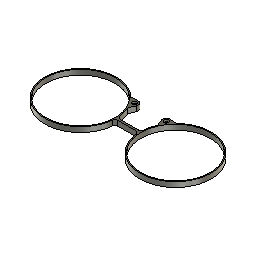
Prop Guard Back v17 (Autodesk Fusion 360 design; units mm, degrees)
Autodesk Fusion 360 part; units mm, degrees
sketch "Sketch1" plane through (0, 0, 0) normal (0, 0, 1) x (1, 0, 0)
  line L0 (25, 40) -> (-25, 40)
  line L1 (-25, 40) -> (-25, -40)
  line L2 (-25, -40) -> (25, -40)
  line L3 (25, -40) -> (25, 40)
  line L4 (25, 40) -> (-25, -40) construction
  line L5 (-25, 40) -> (25, -40) construction
  line L6 (25, 40) -> (46.6506, 52.5)
  line L7 (25, 40) -> (55, 40) construction
  line L8 (0, 40) -> (0, -40)
  line L9 (-25, 0) -> (25, 0)
  line L10 (25, 40) -> (23.5, 42.5981)
  line L11 (23.5, 42.5981) -> (45.1506, 55.0981)
  line L12 (45.1506, 55.0981) -> (46.6506, 52.5)
  line L13 (25, 40) -> (26.5, 37.4019)
  line L14 (26.5, 37.4019) -> (48.1506, 49.9019)
  line L15 (23.5, 42.5981) -> (19, 40)
  line L16 (26.5, 37.4019) -> (25, 36.5359)
  line L17 (48.1506, 49.9019) -> (46.6506, 52.5)
  circle A0 centre (46.6506, 52.5) radius 12
  circle A1 centre (46.6506, 52.5) radius 10
  line L18 (46.6506, 52.5) -> (41.6506, 61.1603)
  line L19 (46.6506, 52.5) -> (55.3109, 57.5)
  line L20 (46.6506, 52.5) -> (51.6506, 43.8397)
  circle A2 centre (46.6506, 52.5) radius 1.5
  line L21 (46.6506, 52.5) -> (51.8468, 55.5)
  line L22 (46.6506, 52.5) -> (43.6506, 57.6962)
  circle A3 centre (-46.6506, 52.5) radius 1.5
  line L23 (-23.5, 42.5981) -> (-45.1506, 55.0981)
  line L24 (-26.5, 37.4019) -> (-48.1506, 49.9019)
  circle A4 centre (-46.6506, 52.5) radius 12
  circle A5 centre (-46.6506, 52.5) radius 10
  line L25 (-26.5, 37.4019) -> (-25, 36.5359)
  line L26 (-23.5, 42.5981) -> (-19, 40)
  circle A6 centre (-46.6506, -52.5) radius 10
  line L27 (-26.5, -37.4019) -> (-48.1506, -49.9019)
  line L28 (-23.5, -42.5981) -> (-45.1506, -55.0981)
  line L29 (-23.5, -42.5981) -> (-19, -40)
  line L30 (-26.5, -37.4019) -> (-25, -36.5359)
  line L31 (23.5, -42.5981) -> (19, -40)
  line L32 (26.5, -37.4019) -> (25, -36.5359)
  line L33 (26.5, -37.4019) -> (48.1506, -49.9019)
  line L34 (23.5, -42.5981) -> (45.1506, -55.0981)
  circle A7 centre (46.6506, -52.5) radius 12
  circle A8 centre (46.6506, -52.5) radius 10
  circle A9 centre (46.6506, -52.5) radius 1.5
  circle A10 centre (-46.6506, -52.5) radius 10
  circle A11 centre (-46.6506, -52.5) radius 12
  line L35 (25, 0) -> (25, -40)
  line L36 (0, 0) -> (0, -9)
  line L37 (0, -9) -> (0, -10.6)
  line L38 (0, -9) -> (0, -7.4)
  line L39 (0, -10.6) -> (14, -10.6)
  line L40 (0, -9) -> (1, -9)
  line L41 (0, -7.4) -> (14, -7.4)
  line L42 (14, -10.6) -> (14, -7.4)
  line L43 (-14, -10.6) -> (-14, -7.4)
  line L44 (0, -7.4) -> (-14, -7.4)
  line L45 (0, -10.6) -> (-14, -10.6)
  line L46 (0, 7.4) -> (-14, 7.4)
  line L47 (-14, 10.6) -> (-14, 7.4)
  line L48 (0, 10.6) -> (-14, 10.6)
  line L49 (0, 10.6) -> (14, 10.6)
  line L50 (0, 7.4) -> (14, 7.4)
  line L51 (14, 10.6) -> (14, 7.4)
  line L52 (19, -40) -> (25.9282, -44)
  line L53 (25, -36.5359) -> (25, -31.5359)
  line L54 (19, -40) -> (16, -40)
  line L55 (14.6699, -37.5) -> (34.8771, -37.5) construction
  circle A12 centre (46.6506, -52.5) radius 35
  circle A13 centre (46.6506, -52.5) radius 34
  circle A14 centre (-46.6506, -52.5) radius 35
  circle A15 centre (-46.6506, -52.5) radius 34
  circle A16 centre (-46.6506, 52.5) radius 35
  circle A17 centre (-46.6506, 52.5) radius 34
  circle A18 centre (46.6506, 52.5) radius 35
  circle A19 centre (46.6506, 52.5) radius 34
  line L56 (46.6506, -52.5) -> (46.6506, 52.5)
  line L57 (46.6506, -52.5) -> (-46.6506, -52.5)
  line L58 (46.6506, -52.5) -> (46.6506, -53.5)
  line L59 (-46.6506, -52.5) -> (-46.6506, -53.5)
  line L60 (-46.6506, -53.5) -> (46.6506, -53.5)
  line L61 (46.6506, -52.5) -> (46.6506, -51.5)
  line L62 (-46.6506, -51.5) -> (46.6506, -51.5)
  line L63 (-46.6506, -52.5) -> (-46.6506, -51.5)
  line L64 (-46.6506, 53.5) -> (46.6506, 53.5)
  line L65 (-46.6506, 51.5) -> (46.6506, 51.5)
  line L66 (46.6506, 0) -> (47.1506, 0)
  line L67 (47.1506, 0) -> (47.1506, -17.5036)
  line L68 (47.1506, 0) -> (47.1506, 17.5036)
  line L69 (46.1506, 0) -> (46.1506, 17.5036)
  line L70 (46.1506, 0) -> (46.1506, -17.5036)
  line L71 (-46.1506, 0) -> (-46.1506, 17.5036)
  line L72 (-47.1506, 0) -> (-47.1506, 17.5036)
  line L73 (-47.1506, 0) -> (-47.1506, -17.5036)
  line L74 (-46.1506, 0) -> (-46.1506, -17.5036)
  line L75 (-47.1506, 0) -> (60, 0)
  line L76 (25, -40) -> (25, -30.5)
  line L77 (25, -30.5) -> (15.5, -30.5)
  circle A20 centre (15.5, -30.5) radius 1.2
  circle A21 centre (15.5, -30.5) radius 3.6
  circle A22 centre (-15.5, -30.5) radius 3.6
  circle A23 centre (-15.5, -30.5) radius 1.2
  line L78 (15.5, -30.5) -> (15.5, -29.3)
  circle A24 centre (15.5, -30.5) radius 2.2
  circle A25 centre (-15.5, -30.5) radius 2.2
  point P0 (-46.6506, -52.5)
  dimension "d1" = 50
  dimension "d2" = 80
  dimension "d4" = 25
  dimension "d5" = 30
  dimension "d6" = 3
  dimension "d7" = 25
  dimension "d8" = 24
  dimension "d9" = 20
  dimension "d10" = 3
  dimension "d11" = 6
  dimension "d13" = 6
  dimension "d23" = 9
  dimension "d24" = 1.6
  dimension "d25" = 1.6
  dimension "d26" = 14
  dimension "d51" = 8
  dimension "d76" = 5
  dimension "d77" = 3
  dimension "d88" = 5
  dimension "d130" = 70
  dimension "d131" = 68
  dimension "d132" = 1
  dimension "d133" = 0.5
  dimension "d140" = 9.5
  dimension "d141" = 9.5
  dimension "d142" = 2.4
  dimension "d143" = 7.2
  dimension "d147" = 4.4
  constraint horizontal L0
  constraint perpendicular L0 L1
  constraint parallel L0 L2
  constraint parallel L1 L3
  constraint coincident L4 L36.start
  constraint coincident L5 L36.start
  constraint coincident L36.start origin
  constraint horizontal L7
  constraint midpoint L0 L8.start
  constraint midpoint L2 L8.end
  constraint midpoint L1 L9.start
  constraint midpoint L3 L9.end
  constraint perpendicular L6 L10
  constraint perpendicular L10 L11
  constraint symmetric L0.start L6 L3.end
  constraint symmetric L6 L10.end L13.end
  constraint symmetric L6 L11.end L14.end
  constraint coincident L0 L15.end
  constraint perpendicular L10 L15
  constraint coincident L3 L16.end
  constraint perpendicular L13 L16
  constraint symmetric L12.end L6 L17.end
  constraint coincident L6.end L12.end
  constraint concentric A0 A1
  constraint coincident A1 L18.end
  constraint parallel L12 L18
  constraint coincident A1 L19.end
  constraint perpendicular L12 L19
  constraint coincident A1 L20.end
  constraint perpendicular L19 L20
  constraint perpendicular L20 L21
  constraint parallel L18 L22
  constraint symmetric L8 L10.end L23.start
  constraint symmetric L8 L11.end L23.end
  constraint symmetric L8 L13.end L24.start
  constraint symmetric L8 L14.end L24.end
  constraint symmetric L8 L15.end L26.end
  constraint symmetric L8 L16.end L25.end
  constraint symmetric L8 A0 A4
  constraint symmetric L8 A1 A5
  constraint symmetric L8 A2 A3
  constraint symmetric L9 L10.end L31.start
  constraint symmetric L9 L11.end L34.end
  constraint symmetric L9 L13.end L32.start
  constraint symmetric L9 L14.end L33.end
  constraint symmetric L9 L15.end L31.end
  constraint symmetric L9 L16.end L32.end
  constraint symmetric L9 A0 A7
  constraint symmetric L9 A1 A8
  constraint symmetric L9 A2 A9
  constraint symmetric L9 L23.start L28.start
  constraint symmetric L9 L23.end L28.end
  constraint symmetric L9 L24.start L27.start
  constraint symmetric L9 L24.end L27.end
  constraint symmetric L9 A3.centre P0
  constraint symmetric L9 A5 A6
  constraint symmetric L9 L25.end L30.end
  constraint symmetric L9 L26.end L29.end
  constraint symmetric L9 A5 A10
  constraint symmetric L9 A4 A11
  constraint perpendicular L9 L36
  constraint parallel L8 L37
  constraint parallel L36 L38
  constraint perpendicular L37 L39
  constraint perpendicular L38 L40
  constraint symmetric L37.end L40 L38.end
  constraint symmetric L39.end L40 L41.end
  constraint symmetric L8 L37.end L39.start
  constraint symmetric L8 L39.end L43.start
  constraint symmetric L8 L38.end L41.start
  constraint symmetric L8 L41.end L43.end
  constraint symmetric L9 L37.end L48.start
  constraint symmetric L9 L39.end L49.end
  constraint symmetric L9 L38.end L46.start
  constraint symmetric L9 L41.end L50.end
  constraint symmetric L9 L43.start L47.start
  constraint symmetric L9 L43.end L46.end
  constraint parallel L34 L52
  constraint parallel L2 L54
  constraint horizontal L55
  constraint concentric A8 A12
  constraint concentric A9 A13
  constraint symmetric L8 A12 A14
  constraint symmetric L8 A13 A15
  constraint symmetric L9 A12 A18
  constraint symmetric L9 A13 A19
  constraint symmetric L9 A14 A16
  constraint symmetric L9 A15 A17
  constraint coincident A7.centre A8.centre
  constraint coincident P0 A6.centre
  constraint perpendicular L57 L58
  constraint symmetric L8 A7.centre P0
  constraint symmetric L8 L58.end L59.end
  constraint symmetric L57 A7.centre A8.centre
  constraint symmetric L57 L58.end L61.end
  constraint symmetric L57 P0 A6.centre
  constraint symmetric L57 L59.end L62.start
  constraint symmetric L9 L58.end L64.end
  constraint symmetric L9 L59.end L64.start
  constraint symmetric L9 L61.end L65.end
  constraint symmetric L9 L62.start L65.start
  constraint midpoint L56 L66.start
  constraint perpendicular L56 L66
  constraint coincident A12 L67.end
  constraint perpendicular L66 L67
  constraint coincident A18 L68.end
  constraint perpendicular L66 L68
  constraint symmetric L56 L66.end L69.start
  constraint symmetric L56 L67.end L70.end
  constraint symmetric L56 L68.end L69.end
  constraint symmetric L8 L66.end L72.start
  constraint symmetric L8 L67.end L73.end
  constraint symmetric L8 L68.end L72.end
  constraint symmetric L8 L69.start L71.start
  constraint symmetric L8 L69.end L71.end
  constraint symmetric L8 L70.end L74.end
  constraint perpendicular L71 L75
  constraint perpendicular L2 L76
  constraint perpendicular L35 L77
  constraint coincident L77.end A20.centre
  constraint concentric A20 A21
  constraint symmetric L8 A20 A23
  constraint symmetric L8 A21 A22
  constraint coincident A20 L78.end
  constraint perpendicular L77 L78
  constraint concentric A20 A24
  constraint symmetric L8 A24 A25
  measures "d1" distance of L1.end L2.end
  measures "d2" distance of L0.end L1.end
  measures "d4" distance of L0.start L6.end
  measures "d5" angle of L6 L7
  measures "d6" distance of L0.start L10.end
  measures "d7" distance of L10.end L11.end
  measures "d8" diameter of A0
  measures "d9" diameter of A1
  measures "d10" diameter of A2
  measures "d11" distance of L6.end L21.end
  measures "d13" distance of L6.end L22.end
  measures "d23" distance of L36.start L36.end
  measures "d24" distance of L36.end L37.end
  measures "d25" distance of L36.end L38.end
  measures "d26" distance of L37.end L39.end
  measures "d51" distance of L31.end L52.end
  measures "d76" distance of L32.end L53.end
  measures "d77" distance of L31.end L54.end
  measures "d88" distance of L31.end L55.start
  measures "d130" diameter of A12
  measures "d131" diameter of A13
  measures "d132" distance of A7.centre L58.end
  measures "d133" distance of L66.start L66.end
  measures "d140" distance of L2.end L76.end
  measures "d141" distance of L76.end L77.end
  measures "d142" diameter of A20
  measures "d143" diameter of A21
  measures "d147" diameter of A24
extrude "Extrude6" add sketch "Sketch1" along normal blind 5 contours L3 L35 A12 A13 L56 | L3 L35 A12 A13 L77 | L2 A12 A13 L77 A21 | A12 A13 L56 L60 | A12 A21 | A12 A21 | L1 L2 A14 A15 A22 | L1 A14 A15 L60 | L2 A12 A13 L62 | A14 A22 | A14 A22 | A12 A13 L57 L60 | A12 A13 L57 L62 | L2 A14 A15 L62 | A14 A15 L57 L60 | A12 A14 L57 L60 | A12 A14 L57 L62 | A14 A15 L57 L62 | A24 | A25
chamfer "Chamfer39" distance 5 angle 45 4 edges at (17.1185, -33.7157, 2.5) (19.0718, -30.9499, 2.5) (-19.0718, -30.9499, 2.5) (-17.1185, -33.7157, 2.5)
chamfer "Chamfer40" distance 2 angle 45 4 edges at (11.6649, -51.5, 2.5) (11.6649, -53.5, 2.5) (-11.6649, -51.5, 2.5) (-11.6649, -53.5, 2.5)
extrude "Extrude7" cut sketch "Sketch1" along normal blind 5 and the other way blind -3 contours A24 | A25
equation "d143 = 3.2 mm + 4 mm"
